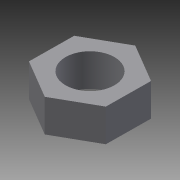
# Autodesk Inventor part: SpanoloAnya
Saved by Autodesk Inventor 2015 (Build 190159000, 159)
## iProperties
Created: 2014-09-09
Part Number: SpanoloAnya
Material: Generic
Document SubType Name: Modeling
Designer: laca
Density: 1 g/cm^3
Appearance: Default
Mass: 2.11302 g
Surface Area: 14.7783 cm^2
Volume: 2.11302 cm^3
Author: laca
Autodesk Inventor part; units mm, degrees
ref_plane "YZ Plane" through (0, 0, 0) normal (1, 0, 0) x (0, 1, 0)
ref_plane "XZ Plane" through (0, 0, 0) normal (0, 1, 0) x (-1, 0, 0)
ref_plane "XY Plane" through (0, 0, 0) normal (0, 0, 1) x (1, 0, 0)
sketch "Sketch1" plane through (0, 0, 0) normal (0, 1, 0) x (-1, 0, 0)
  line L0 (9.5795, 5.4068) -> (9.4722, -5.5927)
  line L1 (9.4722, -5.5927) -> (-0.1073, -10.9995)
  line L2 (-0.1073, -10.9995) -> (-9.5795, -5.4068)
  line L3 (-9.5795, -5.4068) -> (-9.4722, 5.5927)
  line L4 (-9.4722, 5.5927) -> (0.1073, 10.9995)
  line L5 (0.1073, 10.9995) -> (9.5795, 5.4068)
  circle A0 centre (0, 0) radius 6
  circle A1 centre (0, 0) radius 9
  dimension "d0" = 11
  dimension "d1" = 12
  dimension "d8" = 18
  constraints: 12 end point, 3 coincident, 2 centre point, 13 other
  measures "d0" distance of L0.end L1.end
  measures "d1" diameter of A0
  measures "d8" diameter of A1
extrude "Extrusion1" add sketch "Sketch1" along normal blind 8 contours L0 L1 L2 L3 L4 L5 | A1
extrude "Extrusion2" add sketch "Sketch1" against normal blind 4 contours A1
fillet "Fillet1" radius 2 1 edges at (9, -4, 0)
chamfer "Chamfer1" distance 1 angle 45 1 edges at (9, 0, 0)
thread "Thread1" size "M12x1.75" class "6H" standard "ANSI Metric M Profile" full length
chamfer "Chamfer2" distance 1 angle 45 2 edges at (6, -4, 0) (6, 8, 0)
fillet "Fillet3" radius 1 6 edges at (-9.5795, 4, 5.4068) (-9.4722, 4, -5.5927) (0.1073, 4, -10.9995) (-0.1073, 4, 10.9995) (9.4722, 4, 5.5927) (9.5795, 4, -5.4068)
fillet "Fillet4" radius 0.3 12 edges at (9.339, 8, 5.514) (9.5258, 8, 0.0929) (9.4448, 8, -5.3308) (4.8434, 8, -8.2031) (0.1058, 8, -10.8448) (-4.6824, 8, -8.2961) (-9.339, 8, -5.514) (-9.5258, 8, -0.0929) (-9.4448, 8, 5.3308) (-4.8434, 8, 8.2031) (-0.1058, 8, 10.8448) (4.6824, 8, 8.2961)
body "Solid1"
